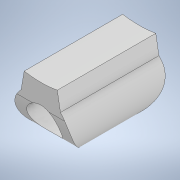
# Autodesk Inventor part: duct_round
Saved by Autodesk Inventor 2020 (Build 240168000, 168)
## iProperties
Created: 2022-09-28
Part Number: duct_round
Material: Generisch
Document SubType Name: Modeling
Designer: sp
Density: 1 g/cm^3
Appearance: Vorgabe
Author: sp
Autodesk Inventor part; units mm, degrees
ref_plane "YZ Plane" through (0, 0, 0) normal (1, 0, 0) x (0, 1, 0)
ref_plane "XZ Plane" through (0, 0, 0) normal (0, 1, 0) x (-1, 0, 0)
ref_plane "XY Plane" through (0, 0, 0) normal (0, 0, 1) x (1, 0, 0)
sketch "Skizze1" plane through (0, 0, 0) normal (0, 0, 1) x (1, 0, 0)
  circle A0 centre (0, 0) radius 5
  circle A1 centre (0, 0) radius 8.5
  dimension "d0" = 10
  dimension "d1" = 17
  constraints: 2 centre point, 2 coincident
  measures "d0" diameter of A0
  measures "d1" diameter of A1
extrude "Extrusion1" add sketch "Skizze1" along normal mid plane 30
sketch "Skizze2" plane through (0, 0, 0) normal (0, 0, 1) x (1, 0, 0)
  line L0 (0, 40.0774) -> (0, -42.4456) construction
  line L1 (-37.8898, 0) -> (75.0495, 0) construction
  circle A0 centre (0, 40) radius 30.5 construction
  circle A1 centre (0, 40) radius 30.5
  circle A2 centre (0, 0) radius 8.5 projected
  line L2 (-4, 7.5) -> (-4, 9.7634)
  line L3 (4, 7.5) -> (4, 9.7634)
  circle A3 centre (0, 0) radius 8.5
  circle A4 centre (0, 40) radius 29
  line L4 (0, 40) -> (5.9896, 6.0311)
  line L5 (5.8214, 6.9852) -> (0, 40)
  line L6 (0, 40) -> (-5.9896, 6.0311)
  point P0 (-5.0358, 11.4406)
  point P1 (-5.9896, 6.0311)
  point P2 (5.9896, 6.0311)
  point P3 (5.0358, 11.4406)
  dimension "d4" = 61
  dimension "d5" = 40
  dimension "d6" = 8
  dimension "d7" = 1.5
  dimension "d8" = 10
  dimension "d9" = 10
  constraints: 14 end point, 6 point on circle, 4 centre point, 4 point on line, 3 vertical, 2 coincident, 2 concentric, 1 collinear, 1 horizontal, 1 other
  measures "d4" diameter of A0
  measures "d5" distance of point (0, 0) A0.centre
  measures "d6" distance between parallel lines of L3 L2
  measures "d7" radial gap between concentric circles of A0 A4
  measures "d8" angle of L4 L0
  measures "d9" angle of L6 L0
extrude "Extrusion2" add sketch "Skizze2" along normal mid plane 30 contours A1 L6 A4 L4 | L2 A2 L6 A1 | A1 L3 A2 L2 | A1 L4 A2 L3 picked at (3.574, 10.751)
sketch "Skizze3" plane through (0, 0, 0) normal (1, 0, 0) x (0, 1, 0)
  line L0 (-8.5, -15) -> (-8.5, 15) projected
  line L1 (-8.5, -15) -> (6.0311, -15) projected
  arc A0 (-8.5, 0) -> (6.0311, -15) centre (5.1952, -1.2713) ccw
  line L2 (6.0311, -15) -> (-8.5, -15)
  line L3 (-8.5, -15) -> (-8.5, 0)
  point P0 (0, 0)
  point P1 (4.3593, -15)
  point P2 (-8.5, -2.5427)
  constraints: 4 end point, 2 point on circle, 1 centre point, 1 collinear, 1 midpoint
extrude "Extrusion3" cut sketch "Skizze3" against normal mid plane 30 contours L0 A0 L1
mirror "Spiegeln1" about plane through (0, 0, 0) normal (0, 0, 1) of "Extrusion3"
